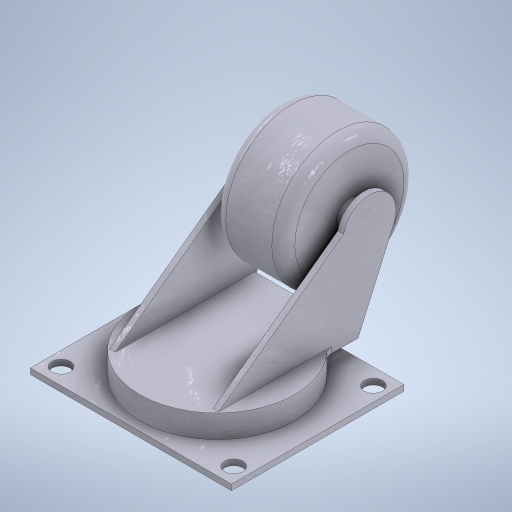
# Autodesk Inventor part: rearaxle
Saved by Autodesk Inventor 2023 (Build 270158000, 158)
## iProperties
Created: 2022-11-29
Part Number: rearaxle
Material: Stainless Steel AISI 440C, Welded
Document SubType Name: Modeling
Designer: kakik
Density: 7.8 g/cm^3
Appearance: Weld - Stainless Steel
Author: kakik
Autodesk Inventor part; units mm, degrees
ref_plane "YZ Plane" through (0, 0, 0) normal (1, 0, 0) x (0, 1, 0)
ref_plane "XZ Plane" through (0, 0, 0) normal (0, 1, 0) x (-1, 0, 0)
ref_plane "XY Plane" through (0, 0, 0) normal (0, 0, 1) x (1, 0, 0)
sketch "Sketch1" plane through (0, 0, 0) normal (0, 1, 0) x (-1, 0, 0)
  line L0 (17.5, 15) -> (-17.5, 15)
  line L1 (-17.5, 15) -> (-17.5, -15)
  line L2 (-17.5, -15) -> (17.5, -15)
  line L3 (17.5, -15) -> (17.5, 15)
  line L4 (17.5, 15) -> (-17.5, -15) construction
  line L5 (-17.5, 15) -> (17.5, -15) construction
  point P0 (0, 0)
  dimension "d0" = 35
  dimension "d1" = 30
  constraints: 12 end point, 2 midpoint, 2 parallel, 1 horizontal, 1 perpendicular
  measures "d0" distance of L2.end L1.end
  measures "d1" distance of L2.end L0.start
extrude "Extrusion1" add sketch "Sketch1" along normal blind 1
sketch "Sketch2" plane through (0, 1, 0) normal (0, 1, 0) x (1, 0, 0)
  line L0 (-17.5, 15) -> (-17.5, -15) projected
  line L1 (-17.5, 0) -> (17.5, 0)
  line L2 (17.5, -15) -> (17.5, 15) projected
  line L3 (-17.5, -15) -> (17.5, -15) projected
  line L4 (0, -15) -> (0, 15)
  line L5 (17.5, 15) -> (-17.5, 15) projected
  point P0 (0, 0)
  point P1 (-15.025, -12.1525)
  point P2 (-15.025, 12.1525)
  point P3 (15.025, -12.1525)
  point P4 (15.025, 12.1525)
  dimension "d11" = 15.025
  dimension "d12" = 12.1525
  constraints: 4 end point, 4 midpoint, 3 symmetric about line
  measures "d11" horizontal distance of point (0, 0) point (-15.025, -12.153)
  measures "d12" vertical distance of point (0, 0) point (-15.025, -12.153)
hole "Hole1" at (-15.025, 1, 12.1525) at (-15.025, 1, -12.1525) at (15.025, 1, -12.1525) at (15.025, 1, 12.1525) direction (0, -1, 0) diameter 3.2 end through all clearance for "Countersunk Flat Head Screw DIN EN ISO 2009" size "M3" standard "DIN"
sketch "Sketch3" plane through (0, 1, 0) normal (0, 1, 0) x (1, 0, 0)
  circle A0 centre (0, 0) radius 13.5
  dimension "d13" = 27
  constraints: 1 centre point, 1 coincident
  measures "d13" diameter of A0
extrude "Extrusion2" add sketch "Sketch3" along normal blind 3
sketch "Sketch4" plane through (0, 4, 0) normal (0, 1, 0) x (1, 0, 0)
  circle A0 centre (0, 0) radius 13.5 projected
  line L0 (17.5, 15) -> (-17.5, 15) projected
  line L1 (-9.5, 15) -> (9.5, 15)
  line L2 (9.5, 15) -> (9.5, 8)
  line L3 (9.5, 8) -> (-9.5, 8)
  line L4 (-9.5, 8) -> (-9.5, 15)
  line L5 (-9.5, 15) -> (9.5, 8) construction
  line L6 (9.5, 15) -> (-9.5, 8) construction
  point P0 (0, 11.5)
  point P1 (0, 8)
  point P2 (-9.5, 9.5917)
  point P3 (9.5, 9.5917)
  dimension "d16" = 19
  dimension "d17" = 7
  constraints: 12 end point, 3 midpoint, 2 parallel, 1 collinear, 1 horizontal, 1 perpendicular, 1 vertical alignment
  measures "d16" distance of L2.end L3.end
  measures "d17" distance of L1.end L2.end
extrude "Extrusion3" add sketch "Sketch4" along normal blind 1
sketch "Sketch5" plane through (9.5, 4, -9.5917) normal (1, 0, 0) x (0, 0, -1)
  line L0 (0, 0) -> (5.4083, 0) projected
  line L1 (5.4083, 0) -> (11.637, 14.1369)
  arc A0 (11.637, 14.1369) -> (2.8827, 16.9336) centre (7.4083, 16) ccw
  line L2 (2.8827, 16.9336) -> (0, 0)
  line L3 (2.8827, 16.9336) -> (-18.8286, 1)
  line L4 (0, 1) -> (-23.0917, 1) projected
  line L5 (0, 1) -> (1.0062, 1)
  line L6 (5.4083, 1) -> (0, 1) projected
  point P0 (-9.5917, -4)
  point P1 (0.1702, 1)
  dimension "d20" = 16
  dimension "d31" = 2
  constraints: 8 end point, 2 point on circle, 2 point on line, 1 centre point, 1 tangent
  measures "d20" vertical distance of L0.end A0.centre
  measures "d31" horizontal distance of A0.centre L0.end
extrude "Extrusion4" add sketch "Sketch5" against normal blind 1
mirror "Mirror1" about plane through (0, 0, 0) normal (1, 0, 0) of "Extrusion4"
fillet "Fillet2" radius 2 2 edges at (-9.5, 4.5, -9.5917) (9.5, 4.5, -9.5917)
sketch "Sketch6" plane through (0, 0, 0) normal (1, 0, 0) x (0, 1, 0)
  arc A0 (18.1369, -21.2287) -> (20.9336, -12.4744) centre (20, -17) ccw projected
  circle A1 centre (20, -17) radius 11.5
  point P0 (0, 0)
  dimension "d25" = 23
  constraints: 1 centre point, 1 coincident
  measures "d25" diameter of A1
extrude "Extrusion5" add sketch "Sketch6" along normal mid plane 12
sketch "Sketch7" plane through (8.5, 4, -9.5917) normal (-1, 0, 0) x (0, 0, 1)
  arc A0 (-2.8827, 16.9336) -> (-11.637, 14.1369) centre (-7.4083, 16) ccw projected
  circle A1 centre (-7.4083, 16) radius 2.3211
  point P0 (9.5917, -4)
  constraints: 1 centre point, 1 coincident
extrude "Extrusion6" add sketch "Sketch7" along normal up to surface (17 mm away)
fillet "Fillet3" radius 2 2 edges at (6, 8.5, -17) (-6, 8.5, -17)
body "Solid1"
